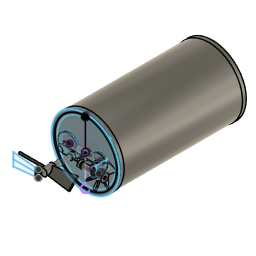
2024_09_30_SubmarineBrick v3 (Autodesk Fusion 360 design; units mm, degrees)
Autodesk Fusion 360 part; units mm, degrees
sketch "Sketch1" plane through (0, 0, 0) normal (0, 1, 0) x (1, 0, 0)
  circle A0 centre (0, 0) radius 50
  circle A1 centre (0, 0) radius 54.3704
  dimension "d1" = 100
  constraint coincident A0.centre A1.centre
  constraint concentric A0 A1
  measures "d1" diameter of A0
extrude "Extrude1" add sketch "Sketch1" along normal blind 200 makes body 1
extrude "Extrude2" add sketch "Sketch1" along normal blind 3 and the other way blind 3 separate body contours A0 makes body 2
sketch "Sketch2" plane through (0, 0, 0) normal (1, 0, 0) x (0, 1, 0)
  line L0 (0, -50) -> (0, 50)
  line L1 (0, 0) -> (0, 50)
  circle A0 centre (0, 50) radius 1.5
  dimension "d6" = 50
  dimension "d7" = 3
  constraint coincident L1.start origin
  constraint parallel L0 L1
  constraint coincident L0.end L1.end
  measures "d6" distance of L1.start L0.end
  measures "d7" diameter of A0
revolve "Revolve1" add sketch "Sketch2" angle 360 about axis through (0, 0, 0) along (0, -1, 0) separate body makes body 3
move_body "Move1" bodies 2 3 to x (1, 0, 0) y (0, 1, 0) z (0, 0, 1) at (0, 5, 0)
copy_body "CopyPasteBodies1" bodies 3 2 makes body 4 makes body 5
move_body "Move2" bodies 4 5 to x (1, 0, 0) y (0, 1, 0) z (0, 0, 1) at (0, 190, 0)
sketch "Sketch3" plane through (0, 0, 0) normal (0, 1, 0) x (1, 0, 0)
  circle A0 centre (0, 0) radius 10 construction
  circle A1 centre (0, 0) radius 4 construction
  line L0 (0, 0) -> (25, 0) construction
  line L1 (0, 0) -> (-25, 0) construction
  circle A2 centre (-25, 0) radius 4
  circle A3 centre (-25, 0) radius 10
  circle A4 centre (25, 0) radius 4
  circle A5 centre (25, 0) radius 10
  dimension "d11" = 20
  dimension "d12" = 8
  dimension "d19" = 25
  dimension "d20" = 25
  constraint coincident A0.centre A1.centre
  constraint horizontal L0
  constraint parallel L0 L1
  constraint coincident L1.end A2.centre
  constraint coincident L0.end A4.centre
  constraint concentric A4 A5
  constraint equal A1 A2
  constraint equal A0 A3
  constraint equal A1 A4
  constraint equal A0 A5
  measures "d11" diameter of A0
  measures "d12" diameter of A1
  measures "d19" distance of A0.centre L0.end
  measures "d20" distance of A0.centre L1.end
extrude "Extrude3" add sketch "Sketch3" along normal blind 10 and the other way blind 2 bodies 2
extrude "Extrude4" cut sketch "Sketch3" along normal blind 50 contours A2 | A4 bodies 2
sketch "Sketch4" plane through (0, 0, 0) normal (0, 1, 0) x (1, 0, 0)
  circle A0 centre (-25, 0) radius 12.831
  circle A1 centre (-8.295, 0) radius 4.746
  line L0 (0, 0) -> (-25, 0)
  line L1 (-8.295, 0) -> (0, 0) construction
  line L2 (0, 0) -> (25, 0)
  line L3 (0, 0) -> (8.295, 0) construction
  circle A2 centre (8.295, 0) radius 4.746
  circle A3 centre (25, 0) radius 12.831
  circle A4 centre (-8.295, 0) radius 3.246
  circle A5 centre (8.295, 0) radius 3.246
  circle A6 centre (-25, 0) radius 16.0344
  point P0 (-25, 0)
  dimension "d21" = -1.5
  dimension "d22" = -1.5
  constraint coincident P0 A0.centre
  constraint coincident A1.centre L0
  constraint coincident A1.centre L1.start
  constraint coincident L0.start L1.end
  constraint coincident L2 L3.end
  constraint equal L1 L3
  constraint coincident L3.end A2.centre
  constraint coincident L2.end A3.centre
  constraint equal A0 A3
  constraint equal A1 A2
  constraint concentric A0 A6
extrude "Extrude5" add sketch "Sketch4" against normal blind 3 separate body contours A0 A1 L0 | A0 A1 L0 | A0 A1 | A2 A3 | L2 A2 A3 | L2 A2 A3 makes body 6 at (-24.0483, 0, -6.6911) makes body 7 at (23.2952, 0, -4.6046)
extrude "Extrude6" add sketch "Sketch4" against normal blind 3 separate body contours A0 A1 L0 | A0 A1 L0 A4 A6 | A0 A1 L0 A4 A6 | A0 A1 L0 | L0 A4 A6 | L0 A4 A6 | A1 L0 A4 A6 | A1 L0 A4 A6 | L0 A4 A6 | L0 A4 A6 | L2 A2 A3 A5 | L2 A2 A3 A5 | L2 A5 | L2 A5 | L2 A2 A3 | L2 A2 A3 makes body 8 at (-3.5726, -2, 0.4726) makes body 9 at (13.0175, -1, -0.4726)
copy_body "CopyPasteBodies2" bodies 8 9 makes body 10 makes body 11
move_body "Move3" bodies 10 11 to x (1, 0, 0) y (0, 1, 0) z (0, 0, 1) at (0, -14, 0)
copy_body "CopyPasteBodies3" bodies 11 makes body 12
move_body "Move4" bodies 12 to x (0, 1, 0) y (-1, 0, 0) z (0, 0, 1) at (-8.705, -25.295, 0)
move_body "Move5" bodies 12 to x (1, 0, 0) y (0, 1, 0) z (0, 0, 1) at (7, -2.9359, 0.6169)
extrude "Extrude7" add sketch "Sketch4" against normal blind 15 contours L0 A4 A6 | L0 A4 A6 | L0 A4 A6 | L0 A4 A6 | L2 A5 | L2 A5 bodies 8 9 10 11
sketch "Sketch5" plane through (15.295, 0, 0) normal (1, 0, 0) x (0, 1, 0)
  circle A0 centre (-19.9359, 0.6169) radius 4.746
  circle A1 centre (-19.9359, 0.6169) radius 2.1538
  constraint concentric A0 A1
extrude "Extrude8" add sketch "Sketch5" along normal blind -6 and the other way blind -35 contours A1 bodies 12
extrude "Extrude9" add sketch "Sketch4" against normal blind 37 separate body contours L0 A4 A6 | L0 A4 A6 | L0 A4 A6 | L0 A4 A6 makes body 13
extrude "Extrude10" add 1 faces at (-9.5563, -17, 2.128) along direction (0, -1, 0) blind 10 on bodies 8 bodies 8 13
sketch "Sketch6" plane through (0, 0, 0) normal (0, 1, 0) x (1, 0, 0)
  line L0 (-25, -5.8814) -> (25, -5.8814)
  arc A0 (25, -5.8814) -> (25, 5.8814) centre (25, 0) ccw
  line L1 (25, 5.8814) -> (-25, 5.8814)
  arc A1 (-25, 5.8814) -> (-25, -5.8814) centre (-25, 0) ccw
  line L2 (-25, 0) -> (25, 0) construction
  line L3 (0, 0) -> (25, 0)
  point P0 (-25, 0)
  point P1 (25, 0)
  constraint tangent L0 A0
  constraint tangent A0 L1
  constraint parallel L0 L1
  constraint tangent L1 A1
  constraint tangent L0 A1
  constraint coincident P1 A0.centre
  constraint parallel L2 L3
  constraint coincident P0 A1.centre
extrude "Extrude11" add sketch "Sketch6" against normal blind 7 separate body makes body 14
move_body "Move6" bodies 14 to x (1, 0, 0) y (0, 1, 0) z (0, 0, 1) at (0, -6, 0)
extrude "Extrude12" add 2 faces at (-4.0667, -3, 0.2358) (12.5113, -3, 0.3971) along direction (0, -1, 0) blind 2 on bodies 8 9 bodies 8 9 12 14
extrude "Extrude13" add sketch "Sketch3" along normal blind 38 and the other way blind 15 separate body contours A2 | A4 makes body 15 at (28.9801, 25.3333, 0.3983) makes body 16 at (-21.0199, 25.3333, 0.3983)
sketch "Sketch7" plane through (0, 2, 0) normal (0, -1, 0) x (1, 0, 0)
  circle A0 centre (-25, 0) radius 10
  circle A1 centre (0, 0) radius 50
  circle A2 centre (25, 0) radius 10
  line L0 (-9.5488, 15.3247) -> (-40.4512, 15.3247)
  line L1 (-40.4512, 15.3247) -> (-40.4512, -15.3247)
  line L2 (-40.4512, -15.3247) -> (-9.5488, -15.3247)
  line L3 (-9.5488, -15.3247) -> (-9.5488, 15.3247)
  line L4 (-9.5488, 15.3247) -> (-40.4512, -15.3247) construction
  line L5 (-40.4512, 15.3247) -> (-9.5488, -15.3247) construction
  line L6 (9.5488, 15.3247) -> (40.4512, 15.3247)
  line L7 (40.4512, 15.3247) -> (40.4512, -15.3247)
  line L8 (40.4512, -15.3247) -> (9.5488, -15.3247)
  line L9 (9.5488, -15.3247) -> (9.5488, 15.3247)
  line L10 (9.5488, 15.3247) -> (40.4512, -15.3247) construction
  line L11 (40.4512, 15.3247) -> (9.5488, -15.3247) construction
  point P0 (-25, 0)
  point P1 (25, 0)
  constraint horizontal L0
  constraint perpendicular L0 L1
  constraint parallel L0 L2
  constraint parallel L1 L3
  constraint coincident L4 P0
  constraint coincident L5 P0
  constraint coincident P0 A0.centre
  constraint horizontal L6
  constraint perpendicular L6 L7
  constraint parallel L6 L8
  constraint parallel L7 L9
  constraint coincident L10 P1
  constraint coincident L11 P1
  constraint coincident P1 A2.centre
  constraint equal L0 L6
  constraint equal L3 L9
extrude "Extrude14" add sketch "Sketch7" against normal blind 45 separate body contours A0 | A2 | L0 L1 L2 L3 | L6 L7 L8 L9 makes body 17 at (-19.8496, 17, 15.3247) makes body 18 at (19.8496, 17, 15.3247)
move_body "Move7" bodies 17 18 to x (1, 0, 0) y (0, 1, 0) z (0, 0, 1) at (0, 20, 0)
chamfer "Chamfer1" distance 5 distance2 3 8 faces at (-19.8496, 37, 15.3247) (-9.5488, 37, -5.1082) (-30.1504, 67, -5.1082) (-40.4512, 37, 5.1082) (19.8496, 67, -5.1082) (19.8496, 37, 15.3247) (40.4512, 37, 5.1082) (9.5488, 37, -5.1082) tangent chain off on bodies 17 18
extrude "Extrude15" add 1 faces at (15.295, -16.0716, 0.8527) along direction (1, 0, 0) blind 6 separate body on bodies 12 makes body 19
move_body "Move8" bodies 19 to x (1, 0, 0) y (0, 1, 0) z (0, 0, 1) at (12, 0, 0)
extrude "Extrude16" add 1 faces at (27.295, -16.0796, 0.9597) along direction (-1, 0, 0) blind 4 on bodies 19 bodies 12 19
sketch "Sketch8" plane through (23.295, 0, 0) normal (-1, 0, 0) x (0, -1, 0)
  circle A0 centre (19.9359, 0.6169) radius 2.1538
  circle A1 centre (19.9359, 0.6169) radius 4.746
  circle A2 centre (19.9359, 0.6169) radius 4.746
  line L0 (19.9359, 0.6169) -> (19.9359, 5.3629)
  line L1 (19.9359, 0.6169) -> (19.9359, -4.1292)
  line L2 (19.9359, -4.1292) -> (13, -4.1292)
  line L3 (13, -4.1292) -> (13, 5.3629)
  line L4 (13, 5.3629) -> (19.9359, 5.3629)
  line L5 (19.9359, 5.3629) -> (19.9359, -4.1292)
  line L6 (13, -5.8814) -> (13, 5.8814)
  circle A3 centre (19.9359, 0.6169) radius 2.1538
  constraint concentric A0 A2
  constraint vertical L0
  constraint coincident A0.centre A1.centre
  constraint coincident A2 L0.end
  constraint vertical L1
  constraint coincident A2 L1.end
  constraint horizontal L2
  constraint vertical L3
  constraint horizontal L4
  constraint vertical L5
  constraint coincident L3.end L6
extrude "Extrude17" add sketch "Sketch8" against normal blind 4 separate body contours A0 A1 A2 L0 L1 L5 A3 | A0 A1 A2 L0 L1 L5 A3 | A1 A2 L2 L3 L4 L6 makes body 20
extrude "Extrude18" cut 1 faces at (33.295, -16.0796, 0.9597) along direction (-1, 0, 0) blind 14 on bodies 12 bodies 12
extrude "Extrude19" add sketch "Sketch8" against normal blind 11 contours A0 A1 A2 L0 L1 L5 A3 | A0 A1 A2 L0 L1 L5 A3 bodies 20
combine "Combine1" operation add target body 6 tool bodies 16
combine "Combine2" operation add target body 7 tool bodies 15
combine "Combine3" operation add target body 14 tool bodies 20
extrude "Extrude20" cut 1 faces at (-23.7663, 38, 1.3296) along direction (0, -1, 0) blind 38 on bodies 6 bodies 6
extrude "Extrude21" cut 1 faces at (23.9962, 38, 2.1865) along direction (0, -1, 0) blind 38 on bodies 7 bodies 7
extrude "Extrude22" add sketch "Sketch3" along normal blind 25 separate body contours A2 | A4 makes body 21 at (-21.0199, 8.3333, 0.3983) makes body 22 at (28.9801, 8.3333, 0.3983)
extrude "Extrude23" add sketch "Sketch3" along normal blind 5 contours A2 | A3 | A4 | A5 bodies 21 22
sketch "Sketch9" plane through (0, 0, 0) normal (0, 1, 0) x (1, 0, 0)
  line L0 (-25.8934, -5.3615) -> (-26.7869, -6.9089)
  line L1 (-26.7869, -6.9089) -> (-25.8934, -8.4564)
  line L2 (-25.8934, -8.4564) -> (-24.1066, -8.4564)
  line L3 (-24.1066, -8.4564) -> (-23.2131, -6.9089)
  line L4 (-23.2131, -6.9089) -> (-24.1066, -5.3615)
  line L5 (-24.1066, -5.3615) -> (-25.8934, -5.3615)
  point P0 (-25, -6.9089)
move_body "Move10" bodies 21 22 to x (1, 0, 0) y (0, 1, 0) z (0, 0, 1) at (0, 5, 0)
extrude "Extrude24" add sketch "Sketch9" along normal blind 1 separate body makes body 23
pattern_circular "C-Pattern1" count 5 over 360 about axis through (-25, 0, 0) along (0, 1, 0) of bodies 23 makes body 24 at (-18.0307, 0, 2.5776) makes body 25 at (-21.4832, 0, -5.3472) makes body 26 at (-28.5168, 0, -5.3472) makes body 27 at (-30.9882, 0, 2.2588)
copy_body "CopyPasteBodies4" bodies 24 27 23 25 26 makes body 28 makes body 29 makes body 30 makes body 31 makes body 32
move_body "Move9" bodies 28 29 30 31 32 to x (1, 0, 0) y (0, 1, 0) z (0, 0, 1) at (50, 0, 0)
copy_body "CopyPasteBodies5" bodies 23 27 26 24 25 30 29 32 28 31 makes body 33 makes body 34 makes body 35 makes body 36 makes body 37 makes body 38 makes body 39 makes body 40 makes body 41 makes body 42
move_body "Move11" bodies 33 34 35 36 37 38 39 40 41 42 to x (1, 0, 0) y (0, 1, 0) z (0, 0, 1) at (0, 4, 0)
combine "Combine4" operation add target body 21 tool bodies 33 34 35 36 37
combine "Combine5" operation add target body 22 tool bodies 38 39 40 42
combine "Combine6" operation add target body 6 tool bodies 23 27 26 25 24
combine "Combine7" operation add target body 7 tool bodies 29 30 32 31 28
combine "Combine8" operation add target body 22 tool bodies 41
move_body "Move12" bodies 21 22 to x (1, 0, 0) y (0, 1, 0) z (0, 0, 1) at (0, 5, 0)
extrude "Extrude25" cut 2 faces at (32.9479, -2, 0.6955) (-17.0521, -2, 0.6955) along direction (0, 1, 0) blind 4 on bodies 2 bodies 2
extrude "Extrude26" cut 2 faces at (-17.0521, 10, 0.6955) (32.9479, 10, 0.6955) along direction (0, -1, 0) blind 2 on bodies 2 bodies 2
extrude "Extrude27" add sketch "Sketch3" along normal blind 8 contours A2 | A4 bodies 2
extrude "Extrude28" cut 1 faces at (52.525, 0, 5.1852) along direction (0, 1, 0) blind 10 on bodies 1 bodies 1
sketch "Sketch10" plane through (0, 2, 0) normal (0, -1, 0) x (1, 0, 0)
  circle A0 centre (25, 0) radius 4
  circle A1 centre (-25, 0) radius 4
  circle A2 centre (0, 0) radius 50
  circle A3 centre (0, 0) radius 46.598
  circle A4 centre (0, 0) radius 54.3704
  circle A5 centre (0, 0) radius 50
  point P0 (0, 50)
  constraint coincident A2.centre A3.centre
  constraint concentric A3 A4
  constraint concentric A3 A5
  constraint coincident A5 P0
extrude "Extrude29" add sketch "Sketch10" against normal blind 6 contours A4 bodies 2
extrude "Extrude30" add sketch "Sketch10" against normal blind 25 contours A2 A5 bodies 2
move_body "Move13" bodies 3 to x (1, 0, 0) y (0, 1, 0) z (0, 0, 1) at (0, 10, 0)
delete_body "RemoveBody1" bodies 5
mirror "Mirror1" about plane through (0, 0, 0) normal (0, 1, 0) of bodies 2 makes body 43
move_body "Move14" bodies 43 to x (1, 0, 0) y (0, 1, 0) z (0, 0, 1) at (0, 208, 0)
extrude "Extrude31" cut 2 faces at (23.9962, 208, 2.1865) (-23.7663, 208, 1.3296) along direction (0, -1, 0) blind 2 on bodies 43 bodies 43
extrude "Extrude32" cut sketch "Sketch3" along normal blind 2 contours A2 | A4 bodies 2
move_body "Move15" bodies 43 1 to x (1, 0, 0) y (0, 1, 0) z (0, 0, 1) at (0, -2, 0)
move_body "Move16" bodies 4 to x (1, 0, 0) y (0, 1, 0) z (0, 0, 1) at (0, -5, 0)
sketch "Sketch11" plane through (34.295, 0, 0) normal (1, 0, 0) x (0, 1, 0)
  circle A0 centre (-19.9359, 0.6169) radius 2.1538
  circle A1 centre (-19.9359, 0.6169) radius 4.746
  circle A2 centre (-19.9359, 0.6169) radius 4.746
  circle A3 centre (-19.9359, 0.6169) radius 6.3698
  point P0 (-19.9359, 5.3629)
  constraint concentric A0 A2
  constraint coincident A2 P0
  constraint concentric A2 A3
extrude "Extrude33" add sketch "Sketch11" along normal blind 11 separate body contours A1 A2 | A3 makes body 44
sketch "Sketch12" plane through (0, 0, 0) normal (0, 1, 0) x (1, 0, 0)
sketch "Sketch13" plane through (45.295, 0, 0) normal (1, 0, 0) x (0, 1, 0)
  circle A0 centre (-19.9359, 0.6169) radius 2.1538
  circle A1 centre (-19.9359, 0.6169) radius 6.3698
  line L0 (-24.0084, 5.5148) -> (-15.8634, 5.5148)
  line L1 (-19.9359, 5.3629) -> (-19.9359, 18.3629)
  line L2 (-19.9359, 18.3629) -> (-28.9694, 18.3629)
  line L3 (-28.9694, 18.3629) -> (-24.0084, 5.5148)
  line L4 (-19.9359, 18.3629) -> (-10.9024, 18.3629)
  line L5 (-15.8634, 5.5148) -> (-10.9024, 18.3629)
  point P0 (-19.9359, 5.3629)
  dimension "d117" = 13
  constraint coincident A1 L0.start
  constraint coincident A1 L0.end
  constraint coincident P0 L1.start
  constraint perpendicular L0 L1
  constraint perpendicular L1 L2
  constraint perpendicular L1 L4
  constraint equal L2 L4
  measures "d117" distance of P0 L1.end
extrude "Extrude34" add sketch "Sketch13" along normal blind 1 and the other way blind 1 separate body contours A1 L0 L1 | A1 L1 L4 L5 | A1 L1 L2 L3 | A1 L0 L1 makes body 45
move_body "Move18" bodies 45 to x (0.707107, -0.707107, 0) y (0.707107, 0.707107, 0) z (0, 0, 1) at (27.3634, 26.1893, 0)
move_body "Move19" bodies 45 to x (1, 0, 0) y (0, 1, 0) z (0, 0, 1) at (-6, 0, 0)
pattern_circular "C-Pattern2" count 5 over 360 about axis through (45.295, -19.9359, 0.6169) along (1, 0, 0) of bodies 45 makes body 46 at (40.962, -32.6622, 5.0177) makes body 47 at (40.962, -28.0539, -10.1266) makes body 48 at (39.0423, -10.6737, -9.2953) makes body 49 at (40.962, -7.0534, 4.5369)
combine "Combine9" operation add target body 44 tool bodies 46 45 49 48 47
move_body "Move20" bodies 44 to x (1, 0, 0) y (0, 1, 0) z (0, 0, 1) at (3, 0, 0)
extrude "Extrude35" add 1 faces at (34.295, -23.7922, 0.2741) along direction (1, 0, 0) blind 5 separate body on bodies 14 makes body 50
extrude "Extrude36" add 1 faces at (23.295, -14.594, 0.6169) along direction (-1, 0, 0) blind 6 separate body on bodies 14 makes body 51
move_body "Move17" bodies 44 to x (1, 0, 0) y (0, 1, 0) z (0, 0, 1) at (3, 0, 0)
combine "Combine12" operation add target body 14 tool bodies 51 50
extrude "Extrude37" add 1 faces at (-7.3437, -37, 1.7432) along direction (0, -1, 0) blind 30 on bodies 8 bodies 8
extrude "Extrude38" add 1 faces at (-4.0787, -27, 0.3971) along direction (0, 1, 0) blind 8 separate body on bodies 8 makes body 52
move_body "Move21" bodies 52 to x (1, 0, 0) y (0, 1, 0) z (0, 0, 1) at (0, -23, 0)
extrude "Extrude39" cut 1 faces at (-4.0787, -27, 0.3971) along direction (0, 1, 0) blind 9 on bodies 8 bodies 8
extrude "Extrude41" add 1 faces at (12.295, -16.0716, 0.3811) along direction (-1, 0, 0) blind 1 on bodies 12 bodies 12 7 14
extrude "Extrude42" cut 1 faces at (9.295, -19.3168, 0.4892) along direction (1, 0, 0) blind 2 on bodies 12 bodies 7 14 12
sketch "Sketch14" plane through (0, -67, 0) normal (0, -1, 0) x (1, 0, 0)
  circle A0 centre (-8.295, 0) radius 3.246
  circle A1 centre (-8.295, 0) radius 3.246
  circle A2 centre (-8.295, 0) radius 4.746
  circle A3 centre (-8.295, 0) radius 5.8814
  line L0 (25, 5.8814) -> (-25, 5.8814)
  constraint concentric A0 A1
  constraint concentric A0 A2
  constraint concentric A1 A3
  constraint tangent A3 L0
extrude "Extrude43" add sketch "Sketch14" against normal blind 15 separate body contours A0 A1 | A2 | A3 makes body 53
sketch "Sketch15" plane through (0, -67, 0) normal (0, -1, 0) x (1, 0, 0)
  circle A0 centre (-8.295, 0) radius 5.8814
  line L0 (-8.295, 5.8814) -> (-8.2658, -5.8814)
  line L1 (-8.295, 0) -> (-48.4846, -0.1)
  line L2 (-48.4846, -0.1) -> (-48.5095, 9.9)
  line L3 (-48.5095, 9.9) -> (-8.295, 5.8814)
  line L4 (-48.4846, -0.1) -> (-48.4598, -10.1)
  line L5 (-48.4598, -10.1) -> (-8.2658, -5.8814)
  dimension "d144" = 10
  dimension "d145" = 10
  constraint coincident A0 L0.start
  constraint coincident A0 L0.end
  constraint coincident A0.centre L1.start
  constraint perpendicular L0 L1
  constraint perpendicular L1 L2
  constraint perpendicular L1 L4
  measures "d144" distance of L1.end L2.end
  measures "d145" distance of L1.end L4.end
extrude "Extrude44" add sketch "Sketch15" along normal blind 1.5 and the other way blind 1.5 separate body contours A0 L0 | A0 L1 L2 L3 | A0 L1 L4 L5 picked at (-9.9003, 1.7252) makes body 54
move_body "Move22" bodies 54 to x (0.999998, 0.00176, 0.000729) y (-0.00176, 0.707107, 0.707105) z (0.000729, -0.707105, 0.707109) at (-0.1179, -19.6092, 47.3821)
move_body "Move23" bodies 54 to x (1, 0, 0) y (0, 1, 0) z (0, 0, 1) at (0, 8, 0)
pattern_circular "C-Pattern3" count 2 over 360 about axis through (-8.295, -67, 0) along (0, -1, 0) of bodies 54 makes body 55
combine "Combine10" operation add target body 53 tool bodies 55 54
extrude "Extrude45" cut 1 faces at (-7.3437, -67, 1.7432) along direction (0, 1, 0) blind 1 on bodies 8 bodies 8
combine "Combine11" operation add target body 8 tool bodies 52
move_body "Move24" bodies 8 53 to x (1, 0, 0) y (0, 1, 0) z (0, 0, 1) at (2, 0, 0)
extrude "Extrude46" add sketch "Sketch4" against normal blind 3 contours A0 A1 L0 | A0 A1 L0 A4 A6 | A0 A1 L0 A4 A6 | A0 A1 L0 | A0 A1 A6 | L0 A4 A6 | L0 A4 A6 picked at (-9.7927, 0.6466) picked at (-9.7927, -0.6466) bodies 6
extrude "Extrude47" add 1 faces at (-2.0787, -42, 0.3971) along direction (0, 1, 0) blind 7 on bodies 8 bodies 8
extrude "Extrude48" cut 1 faces at (-2.0787, -50, 0.3971) along direction (0, 1, 0) blind 5 on bodies 8 bodies 8
move_body "Move25" bodies 53 to x (1, 0, 0) y (0, 1, 0) z (0, 0, 1) at (0, 6, 0)
extrude "Extrude49" cut 1 faces at (-5.3437, -66, 1.7432) along direction (0, 1, 0) blind 7 on bodies 8 bodies 8
named bodies: "BodyCylinder", "FlatCircleBack", "TorusSiliconBack", "TorusSilicon", "FlatCircle", "TorusSiliconFront", "FlatCircleFront", "MotorGearLeft", "MotorGearRight", "BladeRotorFrontal", "GearJoinLateral", "BladeRotorHorizontal", "PieceKeeper", "MotorFrontal", "MotorHorizontal", "MotorMagnetFrontal", "MotorMagnetLateral", "LateralBlade", "FrontalBlade"
